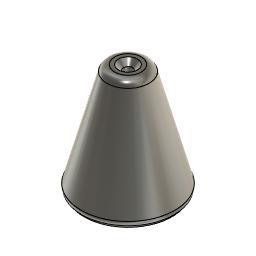
Wobble_Bottom_Transition_Piece (Autodesk Fusion 360 design; units mm, degrees)
Autodesk Fusion 360 part; units mm, degrees
sketch "Sketch1" plane through (0, 0, 0) normal (0, 0, 1) x (1, 0, 0)
  circle A0 centre (0, 0) radius 9.4997
  line L0 (-4.7499, 8.227) -> (-9.4997, 0)
  line L1 (-9.4997, 0) -> (-4.7499, -8.227)
  line L2 (-4.7499, -8.227) -> (4.7499, -8.227)
  line L3 (4.7499, -8.227) -> (9.4997, 0)
  line L4 (9.4997, 0) -> (4.7499, 8.227)
  line L5 (4.7499, 8.227) -> (-4.7499, 8.227)
  circle A1 centre (0, 0) radius 0.9
  dimension "d1" = 16.454
  dimension "d9" = 1.8
  constraint coincident A0.centre A1.centre
  constraint horizontal L3.end A0.centre
  constraint coincident A0 L4.end
  measures "d1" distance of L2 L5
  measures "d9" diameter of A1
extrude "Extrude1" add sketch "Sketch1" along normal blind 21 draft -15 and the other way blind 1 draft 15 contours A0 L4 | A0 L3 | L0 L1 L2 L3 L4 L5 | A0 L5 | A0 L2 | A0 L0 | A0 L1 | A1
fillet "Fillet1" radius 1.6 1 edges at (-3.6107, 1.4005, 21)
extrude "Extrude3" cut sketch "Sketch1" along normal through all and the other way through all contours A1
chamfer "Chamfer2" distance 1 angle 45 3 edges at (-9.1067, -3.5321, -1) (-0.8391, 0.3255, 21) (-0.8391, -0.3255, -1)
fillet "Fillet3" radius 1 1 edges at (-8.8654, 3.4385, -0.0341)
